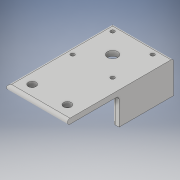
# Autodesk Inventor part: StepperMount
Saved by Autodesk Inventor 2019.4 (Build 234330000, 330)
## iProperties
Created: 2020-12-22
Part Number: StepperMount
Material: Generic
Document SubType Name: Modeling
Designer: Jorian Brusind
Density: 1 g/cm^3
Appearance: Default
Author: Jorian Brusind
Autodesk Inventor part; units mm, degrees
ref_plane "YZ Plane" through (0, 0, 0) normal (1, 0, 0) x (0, 1, 0)
ref_plane "XZ Plane" through (0, 0, 0) normal (0, 1, 0) x (-1, 0, 0)
ref_plane "XY Plane" through (0, 0, 0) normal (0, 0, 1) x (1, 0, 0)
sketch "2020 profile" plane through (0, 0, 0) normal (0, 0, 1) x (1, 0, 0)
  line L0 (8.75, -15.1376) -> (8.75, -9.8624)
  line L1 (2.5, -7.4482) -> (2.5, -3)
  line L2 (4.0732, -9.0732) -> (2.5366, -7.5366)
  line L3 (4.5, -7.125) -> (4.5, -8.8964)
  line L4 (5.8876, -7) -> (4.625, -7)
  line L5 (7, -4.625) -> (7, -5.8876)
  line L6 (7.0366, -5.976) -> (9.774, -8.7134)
  line L7 (8.8964, -4.5) -> (7.125, -4.5)
  line L8 (7.5366, -2.5366) -> (9.0732, -4.0732)
  line L9 (3, -2.5) -> (7.4482, -2.5)
  line L10 (17.5518, -2.5) -> (22, -2.5)
  arc A0 (22.5, -3) -> (22, -2.5) centre (22, -3) ccw
  line L11 (22.5, -3) -> (22.5, -7.4482)
  line L12 (22.4634, -7.5366) -> (20.9268, -9.0732)
  line L13 (20.5, -8.8964) -> (20.5, -7.125)
  line L14 (20.375, -7) -> (19.1124, -7)
  line L15 (18, -5.8876) -> (18, -4.625)
  line L16 (17.875, -4.5) -> (16.1036, -4.5)
  line L17 (15.226, -8.7134) -> (17.9634, -5.976)
  line L18 (19.024, -7.0366) -> (16.2866, -9.774)
  line L19 (16.25, -9.8624) -> (16.25, -15.1376)
  line L20 (16.2866, -15.226) -> (19.024, -17.9634)
  line L21 (19.1124, -18) -> (20.375, -18)
  arc A1 (19.024, -17.9634) -> (19.1124, -18) centre (19.1124, -17.875) ccw
  arc A2 (20.375, -18) -> (20.5, -17.875) centre (20.375, -17.875) ccw
  line L22 (20.5, -17.875) -> (20.5, -16.1036)
  arc A3 (20.9268, -15.9268) -> (20.5, -16.1036) centre (20.75, -16.1036) ccw
  line L23 (20.9268, -15.9268) -> (22.4634, -17.4634)
  arc A4 (22.5, -17.5518) -> (22.4634, -17.4634) centre (22.375, -17.5518) ccw
  line L24 (22.5, -17.5518) -> (22.5, -22)
  line L25 (22, -22.5) -> (17.5518, -22.5)
  line L26 (17.4634, -22.4634) -> (15.9268, -20.9268)
  arc A5 (16.1036, -20.5) -> (15.9268, -20.9268) centre (16.1036, -20.75) ccw
  line L27 (16.1036, -20.5) -> (17.875, -20.5)
  arc A6 (17.875, -20.5) -> (18, -20.375) centre (17.875, -20.375) ccw
  line L28 (18, -20.375) -> (18, -19.1124)
  arc A7 (18, -19.1124) -> (17.9634, -19.024) centre (17.875, -19.1124) ccw
  line L29 (17.9634, -19.024) -> (15.226, -16.2866)
  arc A8 (15.226, -16.2866) -> (15.1376, -16.25) centre (15.1376, -16.375) ccw
  line L30 (15.1376, -16.25) -> (9.8624, -16.25)
  arc A9 (9.8624, -16.25) -> (9.774, -16.2866) centre (9.8624, -16.375) ccw
  line L31 (9.774, -16.2866) -> (7.0366, -19.024)
  circle A10 centre (12.5, -12.5) radius 2
  line L32 (7.125, -20.5) -> (8.8964, -20.5)
  line L33 (9.0732, -20.9268) -> (7.5366, -22.4634)
  arc A11 (9.0732, -20.9268) -> (8.8964, -20.5) centre (8.8964, -20.75) ccw
  line L34 (7.4482, -22.5) -> (3, -22.5)
  arc A12 (7.4482, -22.5) -> (7.5366, -22.4634) centre (7.4482, -22.375) ccw
  arc A13 (7, -20.375) -> (7.125, -20.5) centre (7.125, -20.375) ccw
  line L35 (7, -19.1124) -> (7, -20.375)
  arc A14 (7.0366, -19.024) -> (7, -19.1124) centre (7.125, -19.1124) ccw
  arc A15 (2.5, -22) -> (3, -22.5) centre (3, -22) ccw
  line L36 (2.5, -22) -> (2.5, -17.5518)
  arc A16 (2.5366, -17.4634) -> (2.5, -17.5518) centre (2.625, -17.5518) ccw
  line L37 (2.5366, -17.4634) -> (4.0732, -15.9268)
  arc A17 (4.5, -16.1036) -> (4.0732, -15.9268) centre (4.25, -16.1036) ccw
  line L38 (4.5, -16.1036) -> (4.5, -17.875)
  arc A18 (4.5, -17.875) -> (4.625, -18) centre (4.625, -17.875) ccw
  line L39 (4.625, -18) -> (5.8876, -18)
  line L40 (5.976, -17.9634) -> (8.7134, -15.226)
  arc A19 (5.8876, -18) -> (5.976, -17.9634) centre (5.8876, -17.875) ccw
  arc A20 (8.75, -9.8624) -> (8.7134, -9.774) centre (8.625, -9.8624) ccw
  line L41 (8.7134, -9.774) -> (5.976, -7.0366)
  arc A21 (4.0732, -9.0732) -> (4.5, -8.8964) centre (4.25, -8.8964) ccw
  arc A22 (2.5, -7.4482) -> (2.5366, -7.5366) centre (2.625, -7.4482) ccw
  arc A23 (3, -2.5) -> (2.5, -3) centre (3, -3) ccw
  arc A24 (8.8964, -4.5) -> (9.0732, -4.0732) centre (8.8964, -4.25) ccw
  arc A25 (7.125, -4.5) -> (7, -4.625) centre (7.125, -4.625) ccw
  arc A26 (7.5366, -2.5366) -> (7.4482, -2.5) centre (7.4482, -2.625) ccw
  arc A27 (7, -5.8876) -> (7.0366, -5.976) centre (7.125, -5.8876) ccw
  arc A28 (9.774, -8.7134) -> (9.8624, -8.75) centre (9.8624, -8.625) ccw
  line L42 (9.8624, -8.75) -> (15.1376, -8.75)
  line L43 (15.9268, -4.0732) -> (17.4634, -2.5366)
  arc A29 (17.5518, -2.5) -> (17.4634, -2.5366) centre (17.5518, -2.625) ccw
  arc A30 (15.9268, -4.0732) -> (16.1036, -4.5) centre (16.1036, -4.25) ccw
  arc A31 (20.5, -8.8964) -> (20.9268, -9.0732) centre (20.75, -8.8964) ccw
  arc A32 (22, -22.5) -> (22.5, -22) centre (22, -22) ccw
  point P0 (12.1463, -12.8552)
sketch "2020 Tslot Extrusion" plane through (0, 0, 0) normal (0, 0, 1) x (1, 0, 0)
  line L0 (8.75, -15.1376) -> (8.75, -9.8624)
  line L1 (2.5, -7.4482) -> (2.5, -3)
  line L2 (4.0732, -9.0732) -> (2.5366, -7.5366)
  line L3 (4.5, -7.125) -> (4.5, -8.8964)
  line L4 (5.8876, -7) -> (4.625, -7)
  line L5 (7, -4.625) -> (7, -5.8876)
  line L6 (7.0366, -5.976) -> (9.774, -8.7134)
  line L7 (8.8964, -4.5) -> (7.125, -4.5)
  line L8 (7.5366, -2.5366) -> (9.0732, -4.0732)
  line L9 (3, -2.5) -> (7.4482, -2.5)
  line L10 (17.5518, -2.5) -> (22, -2.5)
  arc A0 (22.5, -3) -> (22, -2.5) centre (22, -3) ccw
  line L11 (22.5, -3) -> (22.5, -7.4482)
  line L12 (22.4634, -7.5366) -> (20.9268, -9.0732)
  line L13 (20.5, -8.8964) -> (20.5, -7.125)
  line L14 (20.375, -7) -> (19.1124, -7)
  line L15 (18, -5.8876) -> (18, -4.625)
  line L16 (17.875, -4.5) -> (16.1036, -4.5)
  line L17 (15.226, -8.7134) -> (17.9634, -5.976)
  line L18 (19.024, -7.0366) -> (16.2866, -9.774)
  line L19 (16.25, -9.8624) -> (16.25, -15.1376)
  line L20 (16.2866, -15.226) -> (19.024, -17.9634)
  line L21 (19.1124, -18) -> (20.375, -18)
  arc A1 (19.024, -17.9634) -> (19.1124, -18) centre (19.1124, -17.875) ccw
  arc A2 (20.375, -18) -> (20.5, -17.875) centre (20.375, -17.875) ccw
  line L22 (20.5, -17.875) -> (20.5, -16.1036)
  arc A3 (20.9268, -15.9268) -> (20.5, -16.1036) centre (20.75, -16.1036) ccw
  line L23 (20.9268, -15.9268) -> (22.4634, -17.4634)
  arc A4 (22.5, -17.5518) -> (22.4634, -17.4634) centre (22.375, -17.5518) ccw
  line L24 (22.5, -17.5518) -> (22.5, -22)
  line L25 (22, -22.5) -> (17.5518, -22.5)
  line L26 (17.4634, -22.4634) -> (15.9268, -20.9268)
  arc A5 (16.1036, -20.5) -> (15.9268, -20.9268) centre (16.1036, -20.75) ccw
  line L27 (16.1036, -20.5) -> (17.875, -20.5)
  arc A6 (17.875, -20.5) -> (18, -20.375) centre (17.875, -20.375) ccw
  line L28 (18, -20.375) -> (18, -19.1124)
  arc A7 (18, -19.1124) -> (17.9634, -19.024) centre (17.875, -19.1124) ccw
  line L29 (17.9634, -19.024) -> (15.226, -16.2866)
  arc A8 (15.226, -16.2866) -> (15.1376, -16.25) centre (15.1376, -16.375) ccw
  line L30 (15.1376, -16.25) -> (9.8624, -16.25)
  arc A9 (9.8624, -16.25) -> (9.774, -16.2866) centre (9.8624, -16.375) ccw
  line L31 (9.774, -16.2866) -> (7.0366, -19.024)
  circle A10 centre (12.5, -12.5) radius 2
  line L32 (7.125, -20.5) -> (8.8964, -20.5)
  line L33 (9.0732, -20.9268) -> (7.5366, -22.4634)
  arc A11 (9.0732, -20.9268) -> (8.8964, -20.5) centre (8.8964, -20.75) ccw
  line L34 (7.4482, -22.5) -> (3, -22.5)
  arc A12 (7.4482, -22.5) -> (7.5366, -22.4634) centre (7.4482, -22.375) ccw
  arc A13 (7, -20.375) -> (7.125, -20.5) centre (7.125, -20.375) ccw
  line L35 (7, -19.1124) -> (7, -20.375)
  arc A14 (7.0366, -19.024) -> (7, -19.1124) centre (7.125, -19.1124) ccw
  arc A15 (2.5, -22) -> (3, -22.5) centre (3, -22) ccw
  line L36 (2.5, -22) -> (2.5, -17.5518)
  arc A16 (2.5366, -17.4634) -> (2.5, -17.5518) centre (2.625, -17.5518) ccw
  line L37 (2.5366, -17.4634) -> (4.0732, -15.9268)
  arc A17 (4.5, -16.1036) -> (4.0732, -15.9268) centre (4.25, -16.1036) ccw
  line L38 (4.5, -16.1036) -> (4.5, -17.875)
  arc A18 (4.5, -17.875) -> (4.625, -18) centre (4.625, -17.875) ccw
  line L39 (4.625, -18) -> (5.8876, -18)
  line L40 (5.976, -17.9634) -> (8.7134, -15.226)
  arc A19 (5.8876, -18) -> (5.976, -17.9634) centre (5.8876, -17.875) ccw
  arc A20 (8.75, -9.8624) -> (8.7134, -9.774) centre (8.625, -9.8624) ccw
  line L41 (8.7134, -9.774) -> (5.976, -7.0366)
  arc A21 (4.0732, -9.0732) -> (4.5, -8.8964) centre (4.25, -8.8964) ccw
  arc A22 (2.5, -7.4482) -> (2.5366, -7.5366) centre (2.625, -7.4482) ccw
  arc A23 (3, -2.5) -> (2.5, -3) centre (3, -3) ccw
  arc A24 (8.8964, -4.5) -> (9.0732, -4.0732) centre (8.8964, -4.25) ccw
  arc A25 (7.125, -4.5) -> (7, -4.625) centre (7.125, -4.625) ccw
  arc A26 (7.5366, -2.5366) -> (7.4482, -2.5) centre (7.4482, -2.625) ccw
  arc A27 (7, -5.8876) -> (7.0366, -5.976) centre (7.125, -5.8876) ccw
  arc A28 (9.774, -8.7134) -> (9.8624, -8.75) centre (9.8624, -8.625) ccw
  line L42 (9.8624, -8.75) -> (15.1376, -8.75)
  line L43 (15.9268, -4.0732) -> (17.4634, -2.5366)
  arc A29 (17.5518, -2.5) -> (17.4634, -2.5366) centre (17.5518, -2.625) ccw
  arc A30 (15.9268, -4.0732) -> (16.1036, -4.5) centre (16.1036, -4.25) ccw
  arc A31 (20.5, -8.8964) -> (20.9268, -9.0732) centre (20.75, -8.8964) ccw
  arc A32 (22, -22.5) -> (22.5, -22) centre (22, -22) ccw
  arc A33 (18, -4.625) -> (17.875, -4.5) centre (17.875, -4.625) ccw
  arc A34 (17.9634, -5.976) -> (18, -5.8876) centre (17.875, -5.8876) ccw
  arc A35 (22.5, -3) -> (22, -2.5) centre (22, -3) ccw
  arc A36 (17.5518, -2.5) -> (17.4634, -2.5366) centre (17.5518, -2.625) ccw
  arc A37 (22.4634, -7.5366) -> (22.5, -7.4482) centre (22.375, -7.4482) ccw
  arc A38 (20.5, -8.8964) -> (20.9268, -9.0732) centre (20.75, -8.8964) ccw
  arc A39 (8.8964, -4.5) -> (9.0732, -4.0732) centre (8.8964, -4.25) ccw
  arc A40 (3, -2.5) -> (2.5, -3) centre (3, -3) ccw
  arc A41 (7.5366, -2.5366) -> (7.4482, -2.5) centre (7.4482, -2.625) ccw
  arc A42 (7.125, -4.5) -> (7, -4.625) centre (7.125, -4.625) ccw
  arc A43 (7, -5.8876) -> (7.0366, -5.976) centre (7.125, -5.8876) ccw
  arc A44 (9.774, -8.7134) -> (9.8624, -8.75) centre (9.8624, -8.625) ccw
  arc A45 (15.1376, -8.75) -> (15.226, -8.7134) centre (15.1376, -8.625) ccw
  arc A46 (4.625, -7) -> (4.5, -7.125) centre (4.625, -7.125) ccw
  arc A47 (4.0732, -9.0732) -> (4.5, -8.8964) centre (4.25, -8.8964) ccw
  arc A48 (5.976, -7.0366) -> (5.8876, -7) centre (5.8876, -7.125) ccw
  arc A49 (20.5, -7.125) -> (20.375, -7) centre (20.375, -7.125) ccw
  arc A50 (19.1124, -7) -> (19.024, -7.0366) centre (19.1124, -7.125) ccw
  arc A51 (16.2866, -9.774) -> (16.25, -9.8624) centre (16.375, -9.8624) ccw
  arc A52 (16.25, -15.1376) -> (16.2866, -15.226) centre (16.375, -15.1376) ccw
  arc A53 (8.7134, -15.226) -> (8.75, -15.1376) centre (8.625, -15.1376) ccw
  arc A54 (17.4634, -22.4634) -> (17.5518, -22.5) centre (17.5518, -22.375) ccw
  line L44 (5.5, -8.8964) -> (5.5, -8)
  line L45 (5.5, -8) -> (5.5251, -8)
  line L46 (5.5251, -8) -> (7.75, -10.2249)
  line L47 (7.75, -10.2249) -> (7.75, -14.7751)
  line L48 (7.75, -14.7751) -> (5.5251, -17)
  line L49 (5.5251, -17) -> (5.5, -17)
  line L50 (5.5, -17) -> (5.5, -16.1036)
  arc A55 (5.5, -16.1036) -> (3.3661, -15.2197) centre (4.25, -16.1036) ccw
  line L51 (3.3661, -15.2197) -> (1.8295, -16.7563)
  arc A56 (1.8295, -16.7563) -> (1.5, -17.5518) centre (2.625, -17.5518) ccw
  line L52 (1.5, -17.5518) -> (1.5, -22)
  arc A57 (1.5, -22) -> (3, -23.5) centre (3, -22) ccw
  line L53 (3, -23.5) -> (7.4482, -23.5)
  arc A58 (7.4482, -23.5) -> (8.2437, -23.1705) centre (7.4482, -22.375) ccw
  line L54 (8.2437, -23.1705) -> (9.7803, -21.6339)
  arc A59 (9.7803, -21.6339) -> (8.8964, -19.5) centre (8.8964, -20.75) ccw
  line L55 (8.8964, -19.5) -> (8, -19.5)
  line L56 (8, -19.5) -> (8, -19.4749)
  line L57 (8, -19.4749) -> (10.2249, -17.25)
  line L58 (10.2249, -17.25) -> (14.7751, -17.25)
  line L59 (14.7751, -17.25) -> (17, -19.4749)
  line L60 (17, -19.4749) -> (17, -19.5)
  line L61 (17, -19.5) -> (16.1036, -19.5)
  arc A60 (16.1036, -19.5) -> (15.2197, -21.6339) centre (16.1036, -20.75) ccw
  line L62 (15.2197, -21.6339) -> (16.7563, -23.1705)
  arc A61 (16.7563, -23.1705) -> (17.5518, -23.5) centre (17.5518, -22.375) ccw
  line L63 (17.5518, -23.5) -> (22, -23.5)
  arc A62 (22, -23.5) -> (23.5, -22) centre (22, -22) ccw
  line L64 (23.5, -22) -> (23.5, -17.5518)
  arc A63 (23.5, -17.5518) -> (23.1705, -16.7563) centre (22.375, -17.5518) ccw
  line L65 (23.1705, -16.7563) -> (21.6339, -15.2197)
  arc A64 (21.6339, -15.2197) -> (19.5, -16.1036) centre (20.75, -16.1036) ccw
  line L66 (19.5, -16.1036) -> (19.5, -17)
  line L67 (19.5, -17) -> (19.4749, -17)
  line L68 (19.4749, -17) -> (17.25, -14.7751)
  line L69 (17.25, -14.7751) -> (17.25, -10.2249)
  line L70 (17.25, -10.2249) -> (19.4749, -8)
  line L71 (19.4749, -8) -> (19.5, -8)
  line L72 (19.5, -8) -> (19.5, -8.8964)
  line L73 (9.8624, -7.75) -> (14.7751, -7.75)
  line L74 (14.7751, -7.75) -> (17, -5.5251)
  line L75 (17, -5.5251) -> (17, -5.5)
  line L76 (17, -5.5) -> (16.1036, -5.5)
  arc A65 (15.2197, -3.3661) -> (16.1036, -5.5) centre (16.1036, -4.25) ccw
  line L77 (15.2197, -3.3661) -> (16.7563, -1.8295)
  line L78 (17.5518, -1.5) -> (22, -1.5)
  arc A66 (17.5518, -1.5) -> (16.7563, -1.8295) centre (17.5518, -2.625) ccw
  line L79 (21.5, -3) -> (21.5, -7.0858)
  line L80 (21.5, -7.0858) -> (20.2197, -8.3661)
  point P0 (12.3493, -11.8573)
  dimension "d10" = 1
  dimension "d11" = 1
  dimension "d12" = 1
  dimension "d13" = 1
  dimension "d14" = 1
  measures "d10" distance between parallel lines of L0 L47
  measures "d11" distance between parallel lines of L42 L73
  measures "d12" distance between parallel lines of L10 L78
  measures "d13" radial gap between concentric circles of A29 A66
  measures "d14" distance between parallel lines of L11 L79
sketch "Sketch1" plane through (0, 0, 0) normal (0, 1, 0) x (-1, 0, 0)
  line L0 (0, 0) -> (42.3, 0)
  line L1 (42.3, 0) -> (42.3, -42.3)
  line L2 (42.3, -42.3) -> (0, -42.3)
  line L3 (0, -42.3) -> (0, 0)
  dimension "d0" = 42.3
  dimension "d1" = 42.3
  constraints: 8 end point, 2 parallel, 1 horizontal, 1 perpendicular
  measures "d0" distance of L1.end L2.end
  measures "d1" distance of L0.end L1.end
extrude "Extrusion1" add sketch "Sketch1" along normal blind 4
sketch "Sketch4" plane through (0, 4, 0) normal (0, 1, 0) x (1, 0, 0)
  circle A0 centre (-21.15, 21.15) radius 4
  line L0 (0, 0) -> (0, 42.3) projected
  line L1 (0, 42.3) -> (-42.3, 42.3) projected
  dimension "d15" = 21.15
  dimension "d16" = 21.15
  dimension "d17" = 8
  constraints: 1 centre point
  measures "d15" distance from line of L0 A0.centre
  measures "d16" distance from line of L1 A0.centre
  measures "d17" diameter of A0
extrude "Extrusion3" cut sketch "Sketch4" against normal blind 5
sketch "Sketch6" plane through (0, 4, 0) normal (0, 1, 0) x (1, 0, 0)
  line L0 (0, 42.3) -> (5, 42.3)
  line L1 (5, 42.3) -> (5, 0)
  line L2 (5, 0) -> (0, 0)
  line L3 (0, 0) -> (0, 42.3)
  point P0 (0, 0)
  dimension "d33" = 5
  dimension "d34" = 42.3
  constraints: 8 end point, 2 parallel, 1 horizontal, 1 perpendicular
  measures "d33" distance of L1.end L2.end
  measures "d34" distance of L0.end L1.end
extrude "Extrusion5" add sketch "Sketch6" against normal blind 25
sketch "Sketch8" plane through (-42.3, 0, 0) normal (0, 0, 1) x (1, 0, 0)
  line L0 (0, 4) -> (47.3, 4) projected
  line L1 (0, 4) -> (47.3, 4)
  line L2 (47.3, 4) -> (47.3, 0)
  line L3 (47.3, 0) -> (0, 0)
  line L4 (0, 0) -> (0, 4)
  point P0 (42.3, 0)
  dimension "d45" = 47.3
  dimension "d46" = 4
  constraints: 8 end point, 2 parallel, 1 horizontal, 1 perpendicular
  measures "d45" distance of L2.end L3.end
  measures "d46" distance of L1.end L2.end
extrude "Extrusion6" add sketch "Sketch8" along normal blind 40
sketch "Sketch9" plane through (0, 4, 0) normal (0, 1, 0) x (1, 0, 0)
  circle A0 centre (-32.3, -30) radius 3
  line L0 (-42.3, 42.3) -> (-42.3, -40) projected
  line L1 (5, -40) -> (-42.3, -40) projected
  circle A1 centre (-5, -30) radius 3
  line L2 (5, 42.3) -> (5, -40) projected
  point P0 (0, 0)
  dimension "d49" = 6
  dimension "d50" = 10
  dimension "d51" = 10
  dimension "d52" = 6
  dimension "d53" = 10
  dimension "d54" = 10
  constraints: 2 centre point
  measures "d49" diameter of A0
  measures "d50" distance from line of L0 A0.centre
  measures "d51" distance from line of L1 A0.centre
  measures "d52" diameter of A1
  measures "d53" distance from line of L1 A1.centre
  measures "d54" distance from line of L2 A1.centre
extrude "Extrusion7" cut sketch "Sketch9" against normal blind 4
sketch "Sketch10" plane through (0, 0, 0) normal (0, -1, 0) x (1, 0, 0)
  circle A0 centre (-21.15, -21.15) radius 4 projected
  circle A1 centre (-21.15, -21.15) radius 11
  line L0 (-42.3, 40) -> (-42.3, -42.3) projected
  line L1 (-42.3, -42.3) -> (0, -42.3)
  line L2 (0, -42.3) -> (0, 0)
  line L3 (0, 0) -> (-42.3, 0)
  line L4 (-42.3, 0) -> (-42.3, -42.3)
  dimension "d57" = 22
  constraints: 8 end point, 2 parallel, 1 centre point, 1 coincident, 1 horizontal, 1 perpendicular
  measures "d57" diameter of A1
extrude "Extrusion8" add sketch "Sketch10" along normal blind 1.75 contours L3 L2 L1 L0
sketch "Sketch5" plane through (0, 4, 0) normal (0, 1, 0) x (1, 0, 0)
  circle A0 centre (-36.65, 5.65) radius 1.5
  line L0 (-42.3, 0) -> (0, 0) projected
  line L1 (-42.3, 42.3) -> (-42.3, 0) projected
  circle A1 centre (-5.65, 5.65) radius 1.5
  circle A2 centre (-36.65, 36.65) radius 1.5
  circle A3 centre (-5.65, 36.65) radius 1.5
  dimension "d20" = 5.65
  dimension "d21" = 5.65
  dimension "d22" = 3
  dimension "d25" = 31
  dimension "d28" = 31
  constraints: 4 centre point, 1 horizontal, 1 vertical, 6 other
  measures "d20" distance from line of L0 A0.centre
  measures "d21" distance from line of L1 A0.centre
  measures "d22" diameter of A0
  measures "d25" distance of A0.centre A1.centre
  measures "d28" distance of A0.centre A2.centre
extrude "Extrusion4" cut sketch "Sketch5" against normal blind 6.75
fillet "Fillet3" radius 2 3 edges at (-42.3, 4, -1.15) (-18.65, 4, -42.3) (-18.65, 4, 40)
fillet "Fillet4" radius 2 1 edges at (-18.65, 0, 0)
fillet "Fillet5" radius 2 1 edges at (-18.65, 0, 40)
fillet "Fillet6" radius 2 4 edges at (0, -21, -21.15) (0, -11.375, -42.3) (0, -1.8748, 0.0039) (0, -11.5, 0)
fillet "Fillet7" radius 2 4 edges at (1, -1.75, -42.3) (-21.15, -1.75, -42.3) (1, -1.75, 0.0157) (-21.15, -1.75, 0.0157)
body "Solid1"
